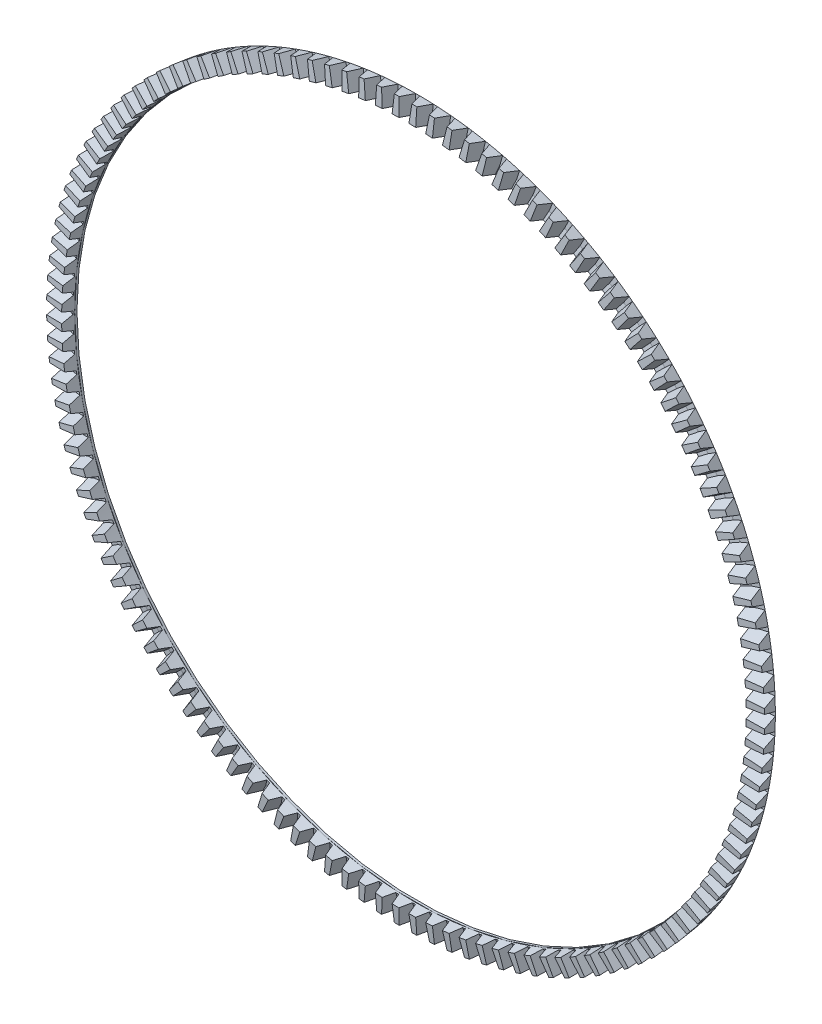
# Autodesk Inventor part: Bevel Gear1
Saved by Autodesk Inventor 2017 (Build 210142000, 142)
## iProperties
Created: 2017-01-10
Part Number: Bevel Gear1
Material: Steel, Mild
Document SubType Name: Modeling
Designer: David Kopala
Categories: <?xml version="1.0" encoding="UTF-16"?> <MemberInstance><Categories><FamilyTemplate><FamilyTemplateParameter ValueType="xs:double" Id="1" ObjectReferenceKey="da_z" ObjectType="kUserParameterObject"/><FamilyTemplateParameter ValueType="xs:double" Id="2" ObjectReferenceKey="da_b" ObjectType="kUserParameterObject"/><FamilyTemplateParameter ValueType="xs:double" Id="3" ObjectReferenceKey="da_beta" ObjectType="kUserParameterObject"/><FamilyTemplateParameter ValueType="xs:double" Id="4" ObjectReferenceKey="da_dae" ObjectType="kUserParameterObject"/><FamilyTemplateParameter ValueType="xs:double" Id="5" ObjectReferenceKey="da_ve" ObjectType="kUserParameterObject"/><FamilyTemplateParameter ValueType="xs:double" Id="6" ObjectReferenceKey="da_omega" ObjectType="kUserParameterObject"/><FamilyTemplateParameter ValueType="xs:string" Id="7" ObjectReferenceKey="EAIAABAAAAAAHwAAAAAAAIAAAAAAAAAA" ObjectType="83914240" SubObjectId="SurfaceGeometry"/></FamilyTemplate><ParamToTemplateMap><ParamToTemplate CategoryParameter="//CategoryParameter[@InternalName='046C89C9-8512-4d59-83FE-43B91F4F132A']" TemplateParameter="1"/><ParamToTemplate CategoryParameter="//CategoryParameter[@InternalName='2552DF32-E462-4b46-AEBF-C6C7768E72AC']" TemplateParameter="2"/><ParamToTemplate CategoryParameter="//CategoryParameter[@InternalName='C9EE641D-15FC-4fae-A226-E94C4372FDD7']" TemplateParameter="3"/><ParamToTemplate><ParamToTemplate CategoryParameter="//CategoryParameter[@InternalName='00B6519A-459B-49c7-AD84-2E56D39A5744']" ConstantValue="0.000000"/></ParamToTemplate><ParamToTemplate><ParamToTemplate CategoryParameter="//CategoryParameter[@InternalName='04B31F0E-C7A6-4894-AA32-9629BEFACF47']" ConstantValue="1.000000"/></ParamToTemplate><ParamToTemplate><ParamToTemplate CategoryParameter="//CategoryParameter[@InternalName='43CBEC2E-7847-49e7-A936-2F7889FCB2D9']" ConstantValue="0.200000"/></ParamToTemplate><ParamToTemplate><ParamToTemplate CategoryParameter="//CategoryParameter[@InternalName='B1EFC894-105D-4ebd-86BF-FA20ED196853']" ConstantValue="0.300000"/></ParamToTemplate><ParamToTemplate><ParamToTemplate CategoryParameter="//CategoryParameter[@InternalName='51175063-3D10-4879-93E8-6246FE8B403D']" ConstantValue="2061532430.657340"/></ParamToTemplate><ParamToTemplate><ParamToTemplate CategoryParameter="//CategoryParameter[@InternalName='A3A52E27-4454-46a9-B0BD-C932399B70AF']" ConstantValue="0.300000"/></ParamToTemplate><ParamToTemplate CategoryParameter="//CategoryParameter[@InternalName='2A200944-5A8C-41ca-B96E-8520D2E510F1']" TemplateParameter="4"/><ParamToTemplate><ParamToTemplate CategoryParameter="//CategoryParameter[@InternalName='1A637F62-92C8-44bc-B81F-10802510B579']" ConstantValue="31.054732"/></ParamToTemplate><ParamToTemplate CategoryParameter="//CategoryParameter[@InternalName='B52DD4BE-6863-48fb-BF58-89EF6F9EC65C']" TemplateParameter="5"/><ParamToTemplate><ParamToTemplate CategoryParameter="//CategoryParameter[@InternalName='3956BFF2-84D2-457d-93C2-9B0613DEBA67']" ConstantValue="1.575781"/></ParamToTemplate><ParamToTemplate CategoryParameter="//CategoryParameter[@InternalName='739CFA02-461B-4bf8-8049-181FCAD8B28F']" TemplateParameter="6"/><ParamToTemplate><ParamToTemplate CategoryParameter="//CategoryParameter[@InternalName='A27E999F-E2CE-4481-8A2A-EBF499C4C3C5']" ConstantValue="0.000000"/></ParamToTemplate><ParamToTemplate><ParamToTemplate CategoryParameter="//CategoryParameter[@InternalName='9E1B4470-B2D3-4ff1-B813-535BB4CDF51A']" ConstantValue="3523220.976809"/></ParamToTemplate><ParamToTemplate><ParamToTemplate CategoryParameter="//CategoryParameter[@InternalName='F8452263-BFF6-458c-9FB1-07C4B99E95CD']" ConstantValue="11397033.805607"/></ParamToTemplate><ParamToTemplate><ParamToTemplate CategoryParameter="//CategoryParameter[@InternalName='3E3BB259-FD49-497f-8171-6EBC954A3479']" ConstantValue="2.000000"/></ParamToTemplate><ParamToTemplate CategoryParameter="//CategoryParameter[@InternalName='27C3BAF2-7550-4e4b-AE2C-0DB134B7D9B7']" TemplateParameter="7"/></ParamToTemplateMap><Category DisplayName="Gear" InternalName="DC85795E-93AB-48d5-8EEE-5A27447B64BD" Mnemonic="Gear"><CategoryParameter DisplayName="z" InternalName="046C89C9-8512-4d59-83FE-43B91F4F132A" Mnemonic="z"/><CategoryParameter DisplayName="b" InternalName="2552DF32-E462-4b46-AEBF-C6C7768E72AC" Mnemonic="b"/><CategoryParameter DisplayName="||b|" InternalName="C9EE641D-15FC-4fae-A226-E94C4372FDD7" Mnemonic="beta"/><CategoryParameter DisplayName="x" InternalName="00B6519A-459B-49c7-AD84-2E56D39A5744" Mnemonic="x"/><CategoryParameter DisplayName="a*" InternalName="04B31F0E-C7A6-4894-AA32-9629BEFACF47" Mnemonic="a"/><CategoryParameter DisplayName="c*" InternalName="43CBEC2E-7847-49e7-A936-2F7889FCB2D9" Mnemonic="c"/><CategoryParameter DisplayName="r|.f|*" InternalName="B1EFC894-105D-4ebd-86BF-FA20ED196853" Mnemonic="rf"/><CategoryParameter DisplayName="E" InternalName="51175063-3D10-4879-93E8-6246FE8B403D" Mnemonic="E"/><CategoryParameter DisplayName="||m|" InternalName="A3A52E27-4454-46a9-B0BD-C932399B70AF" Mnemonic="mi"/><Category DisplayName="BevelGear" InternalName="0C98F69A-0C2B-4791-B2FE-7691BB227E77" Mnemonic="BevelGear"><CategoryParameter DisplayName="d|.ae|" InternalName="2A200944-5A8C-41ca-B96E-8520D2E510F1" Mnemonic="dae"/><CategoryParameter DisplayName="d|.ai|" InternalName="1A637F62-92C8-44bc-B81F-10802510B579" Mnemonic="dai"/><CategoryParameter DisplayName="A|.e|" InternalName="B52DD4BE-6863-48fb-BF58-89EF6F9EC65C" Mnemonic="ve"/><CategoryParameter DisplayName="A|.i|" InternalName="3956BFF2-84D2-457d-93C2-9B0613DEBA67" Mnemonic="vi"/><CategoryParameter DisplayName="||S|" InternalName="739CFA02-461B-4bf8-8049-181FCAD8B28F" Mnemonic="omega"/><CategoryParameter DisplayName="x|.t|" InternalName="A27E999F-E2CE-4481-8A2A-EBF499C4C3C5" Mnemonic="xt"/><CategoryParameter DisplayName="||s||.Flim|" InternalName="9E1B4470-B2D3-4ff1-B813-535BB4CDF51A" Mnemonic="sFlim"/><CategoryParameter DisplayName="||s||.Hlim|" InternalName="F8452263-BFF6-458c-9FB1-07C4B99E95CD" Mnemonic="sHlim"/><CategoryParameter DisplayName="type" InternalName="3E3BB259-FD49-497f-8171-6EBC954A3479" Mnemonic="type"/><CategoryParameter DisplayName="PitchDiameter" InternalName="27C3BAF2-7550-4e4b-AE2C-0DB134B7D9B7" Mnemonic="IDS_PITCHDIAM"/></Category></Category></Categories></MemberInstance>
Mass: 60.9118 g
Surface Area: 34.3074 cm^2
Volume: 7.7496 cm^3
Density: 7.86 g/cm^3
Appearance: Steel
CustomPartVersion: 1
Author: David Kopala
Autodesk Inventor part; units mm, degrees
ref_plane "Mesh Plane2" through (0, 0, 0) normal (0.9996988, 0.0245412, 0) x (0, 0, 1)
sketch "Teeth Body Sketch" plane through (0, 0, 0) normal (1, 0, 0) x (0, 1, 0)
  line L0 (0, 0) -> (162.2052, -22.0773) construction
  line L1 (162.2052, -22.0773) -> (162.8556, -16.5273)
  line L2 (162.8556, -16.5273) -> (0, 0) construction
  line L3 (162.56, -19.05) -> (0, 0) construction
  line L4 (154.6535, -21.0494) -> (155.2737, -15.7578)
  line L5 (162.2052, -22.0773) -> (154.6535, -21.0494)
  line L6 (162.8556, -16.5273) -> (155.2737, -15.7578)
  line L7 (0, -32.5137) -> (0, 36.1422) projected
  line L8 (0, -19.05) -> (162.8556, -19.05) construction
  dimension "d0" = 325.12
  dimension "d1" = 324.4105
  dimension "d2" = 325.7113
  dimension "d3" = 7.62
  dimension "d4" = 16.5273
  constraints: 16 end point, 4 point on line, 3 perpendicular, 2 collinear, 1 horizontal alignment, 1 vertical alignment
  measures "d0" diameter of L3.start L7
  measures "d1" diameter of L0.end L7
  measures "d2" diameter of L1.end L7
  measures "d3" distance between parallel lines of L1 L4
  measures "d4" vertical distance of L1.end L0.start
revolve "Teeth Body" add sketch "Teeth Body Sketch" angle 360 about axis through (0, 0, 0) along (0, 0, 1)
ref_plane "Tooth Plane" through (0, 162.56, -19.05) normal (0, -0.9932035, 0.116391) x (1, 0, 0)
sketch "Start Sketch" plane through (0, 162.56, -19.05) normal (0, -0.9932035, 0.116391) x (1, 0, 0)
  line L0 (0, -1659.5994) -> (0, 329.2549) projected
  arc A0 (-0.7236, -3.7185) -> (-3.4774, 4.2121) centre (-454.1845, -156.7289) ccw
  arc A1 (3.4774, 4.2121) -> (0.7236, -3.7185) centre (454.1845, -156.7289) ccw
  line L1 (-0.7236, -3.7185) -> (0.7236, -3.7185)
  arc A2 (3.4774, 4.2121) -> (-3.4774, 4.2121) centre (0, -1396.6712) ccw
  dimension "d7" = 478.5801
  dimension "d8" = 454.1845
  dimension "d9" = 1239.9423
  dimension "d57" = 1400.8876
  dimension "d58" = 1392.9526
  constraints: 6 point on circle, 3 centre point, 3 symmetric about line, 2 end point, 1 coincident, 1 perpendicular, 1 other
  measures "d7" radius of A0
  measures "d8" horizontal distance of point (0, -1396.671) A0.centre
  measures "d9" vertical distance of point (0, -1396.671) A0.centre
  measures "d57" radius of A2
  measures "d58" distance from line of A2.centre L1
sketch "End Sketch" plane through (0, 154.7143, -18.1306) normal (0, -0.9932035, 0.116391) x (1, 0, 0)
  line L0 (0, -1579.1534) -> (0, 314.8004) projected
  arc A0 (-0.6894, -2.1461) -> (-3.313, 5.4097) centre (-432.7182, -147.9247) ccw
  arc A1 (3.313, 5.4097) -> (0.6894, -2.1461) centre (432.7182, -147.9247) ccw
  line L1 (-0.6894, -2.1461) -> (0.6894, -2.1461)
  arc A2 (3.313, 5.4097) -> (-3.313, 5.4097) centre (0, -1329.263) ccw
  dimension "d12" = 455.9608
  dimension "d15" = 432.7182
  dimension "d16" = 1181.3383
  dimension "d59" = 1334.6768
  dimension "d60" = 1327.1168
  constraints: 6 point on circle, 3 centre point, 3 symmetric about line, 2 end point, 1 coincident, 1 other
  measures "d12" radius of A0
  measures "d15" horizontal distance of A0.centre point (0, -1329.263)
  measures "d16" vertical distance of A0.centre point (0, -1329.263)
  measures "d59" radius of A2
  measures "d60" distance from line of A2.centre L1
loft "Loft" cut profiles "Start Sketch", "End Sketch"
pattern_circular "Circular Pattern" count 128 over 360 about axis through (0, 0, 0) along (0, 0, 1) of "Loft"
ref_plane "End Plane" through (0, 154.7143, -18.1306) normal (0, -0.9932035, 0.116391) x (1, 0, 0)
sketch3d "3D Sketch Right"
ref_plane "End Plane Right" through (-2.8443, 154.6881, -18.1306) normal (0.0182595, -0.9930356, 0.116391) x (0.999831, 0.0183845, 0)
sketch "End Sketch Right" plane through (-2.8443, 154.6881, -18.1306) normal (0.0182595, -0.9930356, 0.116391) x (0.999831, 0.0183845, 0)
  arc A0 (-0.6894, -2.1461) -> (-3.313, 5.4097) centre (-432.7182, -147.9247) ccw
  line L0 (0, -1606.514) -> (0, 321.4866) projected
  arc A1 (3.313, 5.4097) -> (0.6894, -2.1461) centre (432.7182, -147.9247) ccw
  line L1 (-0.6894, -2.1461) -> (0.6894, -2.1461)
  arc A2 (3.313, 5.4097) -> (-3.313, 5.4097) centre (0, -1329.263) ccw
  dimension "d70" = 432.7182
  dimension "d71" = 1181.3383
  dimension "d72" = 455.9608
  dimension "d73" = 1327.1168
  dimension "d74" = 1334.6768
  constraints: 6 point on circle, 3 centre point, 3 symmetric about line, 2 end point, 1 coincident, 1 perpendicular, 1 other
  measures "d70" horizontal distance of A2.centre A0.centre
  measures "d71" vertical distance of point (0, -1329.263) A0.centre
  measures "d72" radius of A0
  measures "d73" distance from line of point (0, -1329.263) L1
  measures "d74" radius of A2
feature "Loft Right" [suppressed]
pattern_circular "Circular Pattern Right" [suppressed]
sketch3d "3D Sketch Left"
ref_plane "End Plane Left" through (2.8542, 154.6881, -18.1616) normal (-0.0183222, -0.9930114, 0.1165871) x (0.9998298, -0.018448, 0)
sketch "End Sketch Left" plane through (2.8542, 154.6881, -18.1616) normal (-0.0183222, -0.9930114, 0.1165871) x (0.9998298, -0.018448, 0)
  line L0 (0, -1606.4962) -> (0, 321.5301) projected
  arc A0 (-0.6894, -2.1153) -> (-3.313, 5.4405) centre (-432.7182, -147.8939) ccw
  arc A1 (3.313, 5.4405) -> (0.6894, -2.1153) centre (432.7182, -147.8939) ccw
  line L1 (-0.6894, -2.1153) -> (0.6894, -2.1153)
  ellipse E0 centre (0, -15.6504) end of major axis (155.2737, -15.6504) minor radius 18.1029 projected
  arc A2 (3.313, 5.4405) -> (-3.313, 5.4405) centre (0, -1329.2322) ccw
  dimension "d56" = 18.1029
  dimension "d30" = 455.9608
  dimension "d31" = 432.7182
  dimension "d32" = 1181.3383
  dimension "d61" = 1334.6768
  dimension "d62" = 1327.1168
  constraints: 6 point on circle, 3 centre point, 3 symmetric about line, 2 end point, 1 coincident, 2 other
  measures "d30" radius of A0
  measures "d31" horizontal distance of point (0, -1329.232) A0.centre
  measures "d32" vertical distance of A0.centre point (0, -1329.232)
  measures "d61" radius of A2
  measures "d62" distance from line of point (0, -1329.232) L1
feature "Loft Left" [suppressed]
pattern_circular "Circular Pattern Left" [suppressed]
sketch "Body Sketch" plane through (0, 0, 0) normal (1, 0, 0) x (0, 1, 0)
  line L0 (0, -32.5137) -> (0, 36.1422) projected
  line L1 (162.2052, -22.0773) -> (154.6535, -21.0494) projected
  line L2 (154.6535, -21.0494) -> (0, -21.0494)
  line L3 (162.2052, -22.0773) -> (0, -22.0773)
  constraints: 4 end point, 2 perpendicular, 2 point on line
revolve "Fix Body" add sketch "Body Sketch" angle 360 about axis through (0, 0, 0) along (0, 0, 1)
sketch "Sketch6" plane through (0, 0, 0) normal (1, 0, 0) x (0, 1, 0)
  line L0 (162.56, -19.05) -> (0, 0) projected
  line L1 (0, -32.5137) -> (0, 36.1422) projected
surface revolve "Pitch Diameter" sketch "Sketch6" angle 360 about axis through (0, 0, 0) along (0, 0, 1) shown no curves L0
sketch "Sketch8" plane through (0, 0, -21.0494) normal (0, 0, 1) x (1, 0, 0)
  point P0 (0, 0)
sketch "Sketch9" plane through (0, 0, -21.0494) normal (0, 0, 1) x (1, 0, 0)
  circle A0 centre (0, 0) radius 154.6479
  dimension "d92" = 309.2958
  constraints: 1 centre point, 1 coincident
  measures "d92" diameter of A0
extrude "Extrusion1" cut sketch "Sketch9" against normal through all
sketch "Sketch10" plane through (154.5138, 8.2822, -20.3494) normal (0.3076793, 0.0151153, 0.95137) x (0.9500072, 0.0509222, -0.3080476)
  ellipse E0 centre (-146.6787, -0.0678) end of major axis (-145.9899, 162.136) minor radius 154.3172 (7.6305, -1.6732) -> (7.6385, 0.2271) ccw projected
  point P0 (-153.4795, -0.0389)
  constraints: 2 other
equation "\"d0\" = da_de"
equation "\"d1\" = da_dfe"
equation "\"d2\" = da_dae"
equation "\"d3\" = da_b"
equation "\"d4\" = da_ve"
equation "\"d7\" = fd_rr"
equation "\"d8\" = fd_x"
equation "\"d9\" = fd_y"
equation "\"d57\" = 0.5 * fd_dva + 0.3 * da_he"
equation "\"d58\" = 0.5 * fd_dva - 1.12 * da_he"
equation "\"da_teethtype\" = 0"
equation "\"da_b\" = 7.62"
equation "\"da_de\" = 325.12"
equation "\"da_dae\" = 325.71127"
equation "\"da_dfe\" = 324.41048"
equation "\"da_le\" = 163.6724"
equation "\"da_omega\" = 90deg"
equation "\"da_beta\" = 0"
equation "\"da_delta\" = 83.316136deg"
equation "\"da_alpha\" = 20deg"
equation "\"da_he\" = 5.588"
equation "\"da_ve\" = 16.52726"
equation "\"da_zv\" = 1099.741093"
equation "\"fd_loft\" = da_b + 0.05 * da_he"
equation "\"fd_x\" = fd_x1 + fd_x2"
equation "\"fd_y\" = fd_y1 - fd_y2"
equation "\"fd_dd\" = fd_dva - 0.8 * da_he"
equation "\"da_dvw\" = 2793.34238"
equation "\"d11\" = fd_loft"
equation "\"da_dm\" = 317.55179"
equation "\"da_x\" = 0"
equation "\"da_m\" = 2.54"
equation "\"d50\" = da_omega"
equation "\"fd_rr\" = 478.580124"
equation "\"fd_dva\" = 2798.422376"
equation "\"fd_x1\" = 1.994911"
equation "\"fd_x2\" = 452.189593"
equation "\"fd_y1\" = 1396.669763"
equation "\"fd_y2\" = 156.727493"
body "Solid1"
body "Srf1"
